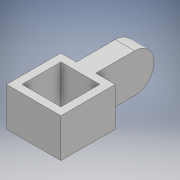
# Autodesk Inventor part: 軸滑塊
Saved by Autodesk Inventor 2017 (Build 210142000, 142)
## iProperties
Part Number: 軸滑塊
Material: 一般
Document SubType Name: Modeling
Designer: Brian
Density: 1 g/cm^3
Appearance: 預設
Author: Brian
Autodesk Inventor part; units mm, degrees
ref_plane "YZ Plane" through (0, 0, 0) normal (1, 0, 0) x (0, 1, 0)
ref_plane "XZ Plane" through (0, 0, 0) normal (0, 1, 0) x (-1, 0, 0)
ref_plane "XY Plane" through (0, 0, 0) normal (0, 0, 1) x (1, 0, 0)
sketch "草圖1" plane through (0, 0, 0) normal (0, 0, 1) x (1, 0, 0)
  line L0 (-5, -5) -> (5, -5)
  line L1 (5, -5) -> (5, 5)
  line L2 (5, 5) -> (-5, 5)
  line L3 (-5, 5) -> (-5, -5)
  line L4 (-5, -5) -> (5, 5) construction
  line L5 (5, -5) -> (-5, 5) construction
  line L6 (-7, 7) -> (7, 7)
  line L7 (7, 7) -> (7, -7)
  line L8 (7, -7) -> (-7, -7)
  line L9 (-7, -7) -> (-7, 7)
  point P0 (0, 0)
  dimension "d0" = 10
  dimension "d1" = 10
  dimension "d2" = 2
  constraints: 20 end point, 4 parallel, 2 midpoint, 2 perpendicular, 1 horizontal, 3 other
  measures "d0" distance of L1.end L2.end
  measures "d1" distance of L0.end L1.end
  measures "d2" distance between parallel lines of L3 L9
extrude "擠出1" add sketch "草圖1" along normal blind 10
sketch "草圖2" plane through (-7, 7, 0) normal (0, 1, 0) x (1, 0, 0)
  line L0 (2, -10) -> (12, -10) projected
  line L1 (12, 0) -> (2, 0) projected
  line L2 (4, -10) -> (9, -10)
  line L3 (9, -10) -> (9, 0)
  line L4 (9, 0) -> (4, 0)
  line L5 (4, 0) -> (4, -10)
  line L6 (14, 0) -> (14, -10) projected
  point P0 (7, 0)
  dimension "d5" = 5
  dimension "d6" = 5
  constraints: 8 end point, 2 parallel, 2 point on line, 1 horizontal, 1 perpendicular
  measures "d5" distance between parallel lines of L5 L3
  measures "d6" distance between parallel lines of L6 L3
extrude "擠出2" add sketch "草圖2" along normal blind 15
fillet "圓角1" radius 5 2 edges at (-0.5, 22, 10) (-0.5, 22, 0)
